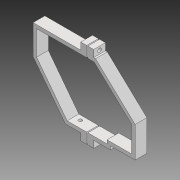
# Autodesk Inventor part: proto_clamp
Saved by Autodesk Inventor 2020 (Build 240168000, 168)
## iProperties
Created: 2021-02-05
Part Number: proto_clamp
Material: Generic
Document SubType Name: Modeling
Designer: DDeGo
Density: 1 g/cm^3
Appearance: Default
Author: DDeGo
Autodesk Inventor part; units mm, degrees
ref_plane "YZ Plane" through (0, 0, 0) normal (1, 0, 0) x (0, 1, 0)
ref_plane "XZ Plane" through (0, 0, 0) normal (0, 1, 0) x (-1, 0, 0)
ref_plane "XY Plane" through (0, 0, 0) normal (0, 0, 1) x (1, 0, 0)
sketch "Sketch1" plane through (0, 0, 0) normal (0, 0, 1) x (1, 0, 0)
  line L0 (53.1863, 0) -> (87, -31.7003)
  line L1 (87, -31.7003) -> (87, -58)
  line L2 (87, -58) -> (66, -58)
  line L3 (66, -58) -> (66, -61)
  line L4 (66, -61) -> (27.5175, -61)
  line L5 (27.5175, -61) -> (0, -25.0156)
  line L6 (0, -25.0156) -> (0, 0)
  line L7 (0, 0) -> (53.1863, 0)
  line L8 (52, -3) -> (84, -33)
  line L9 (84, -33) -> (84, -55)
  line L10 (84, -55) -> (63, -55)
  line L11 (63, -55) -> (63, -58)
  line L12 (63, -58) -> (29, -58)
  line L13 (29, -58) -> (3, -24)
  line L14 (3, -24) -> (3, -3)
  line L15 (3, -3) -> (52, -3)
  dimension "d0" = 3
  dimension "d2" = 52
  dimension "d3" = 55
  dimension "d4" = 21
  dimension "d7" = 81
  dimension "d8" = 22
  dimension "d9" = 21
  dimension "d10" = 49
  dimension "d11" = 34
  constraints: 32 end point, 6 perpendicular, 2 parallel, 1 horizontal, 7 other
  measures "d0" distance between parallel lines of L14 L6
  measures "d2" distance between parallel lines of L10 L15
  measures "d3" distance between parallel lines of L15 L12
  measures "d4" distance between parallel lines of L11 L9
  measures "d7" distance between parallel lines of L14 L9
  measures "d8" distance of L8.end L9.end
  measures "d9" distance of L13.end L14.end
  measures "d10" distance of L14.end L8.start
  measures "d11" distance of L11.end L12.end
extrude "Extrusion1" add sketch "Sketch1" along normal blind 10
sketch "Sketch2" plane through (27.5175, -61, 0) normal (0, -1, 0) x (1, 0, 0)
  circle A0 centre (6.2738, 4) radius 1.5 projected
  point P0 (-27.5175, 0)
extrude "Extrusion2" cut sketch "Sketch2" against normal blind 10
sketch "Sketch3" plane through (0, 0, 10) normal (0, 0, 1) x (1, 0, 0)
  line L0 (45.6423, 2.3043) -> (46.6423, 2.3043)
  line L1 (46.6423, 2.3043) -> (46.6423, -66.739)
  line L2 (46.6423, -66.739) -> (45.6423, -66.739)
  line L3 (45.6423, -66.739) -> (45.6423, 2.3043)
  point P0 (0, 0)
  dimension "d14" = 1
  constraints: 8 end point, 2 parallel, 1 horizontal, 1 perpendicular
  measures "d14" distance of L0.start L0.end
extrude "Extrusion3" cut sketch "Sketch3" against normal through all
sketch "Sketch4" plane through (0, 0, 10) normal (0, 0, 1) x (1, 0, 0)
  line L0 (45.6423, 0) -> (0, 0) projected
  line L1 (45.6423, 0) -> (40.6423, 0)
  line L2 (40.6423, 0) -> (40.6423, 6)
  line L3 (40.6423, 6) -> (45.6423, 6)
  line L4 (45.6423, 6) -> (45.6423, 0)
  line L5 (53.1863, 0) -> (46.6423, 0) projected
  line L6 (46.6423, 0) -> (51.6423, 0)
  line L7 (51.6423, 0) -> (51.6423, 6)
  line L8 (51.6423, 6) -> (46.6423, 6)
  line L9 (46.6423, 6) -> (46.6423, 0)
  line L10 (45.6423, -61) -> (45.6423, -58) projected
  line L11 (45.6423, -61) -> (40.6423, -61)
  line L12 (40.6423, -61) -> (40.6423, -67)
  line L13 (40.6423, -67) -> (45.6423, -67)
  line L14 (45.6423, -67) -> (45.6423, -61)
  line L15 (46.6423, -61) -> (51.6423, -61)
  line L16 (51.6423, -61) -> (51.6423, -67)
  line L17 (51.6423, -67) -> (46.6423, -67)
  line L18 (46.6423, -67) -> (46.6423, -61)
  dimension "d17" = 6
  dimension "d18" = 5
  constraints: 32 end point, 8 parallel, 5 equal length, 4 horizontal, 4 perpendicular, 4 point on line
  measures "d17" distance of L6.end L7.end
  measures "d18" distance of L2.end L3.end
extrude "Extrusion4" add sketch "Sketch4" against normal up to surface (10 mm away)
sketch "Sketch5" plane through (40.6423, -67, 10) normal (-1, 0, 0) x (0, 0, 1)
  line L0 (0, 0) -> (-10, 0) projected
  line L1 (-5, 0) -> (-5, 73) construction
  line L2 (0, 73) -> (-10, 73) projected
  circle A0 centre (-5, 70) radius 1.6
  circle A1 centre (-5, 3) radius 1.6
  point P0 (-10, 67)
  dimension "d21" = 3
  dimension "d22" = 3
  dimension "d23" = 3.2
  constraints: 2 centre point, 2 end point, 2 midpoint, 2 point on line, 1 equal radius
  measures "d21" distance from line of L2 A0.centre
  measures "d22" distance from line of L0 A1.centre
  measures "d23" diameter of A0
extrude "Extrusion5" cut sketch "Sketch5" against normal through all
body "Solid1"
